Autodesk Fusion 360 part; units mm, degrees
note: some values were not read from the file. Set by a fixed rule: the direction of a hole.
(part 10 of 10)
extrude "Extrusion2" add sketch "Skizze2" along normal blind 3.2 separate body contours L4 L5 L6 L7 makes body 2
extrude "Extrusion3" add sketch "Skizze2" along normal blind 1.6 separate body contours L0 L1 L2 L3 L8 L11 L12 L15 L16 L19 L20 L21 L34 L37 makes body 3
move_face "Fläche verschieben1" by (1.6, 0, 0) 1 faces at (1.6, 64.3467, 26.67) on bodies 1
hole "Bohrung1" at (0, 3.81, 76.2) at (0, 96.52, 76.2) at (0, 96.52, 3.81) at (0, 3.81, 3.81) direction (1, 0, 0) diameter 3 depth 1.6 tip angle 180 bodies 3
hidden bodies 1
named bodies: "Leiterplatte", "Rahmen"
